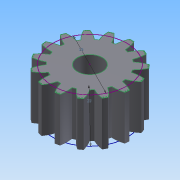
# Autodesk Inventor part: Spur Gear1
Saved by Autodesk Inventor 2015 (Build 190159000, 159)
## iProperties
Created: 2014-09-02
Part Number: Spur Gear1
Material: Steel
Document SubType Name: Modeling
Designer: shohei
Categories: <?xml version="1.0" encoding="UTF-16"?> <MemberInstance><Categories><FamilyTemplate><FamilyTemplateParameter ValueType="xs:double" Id="1" ObjectReferenceKey="da_z" ObjectType="kUserParameterObject"/><FamilyTemplateParameter ValueType="xs:double" Id="2" ObjectReferenceKey="da_b" ObjectType="kUserParameterObject"/><FamilyTemplateParameter ValueType="xs:double" Id="3" ObjectReferenceKey="da_beta" ObjectType="kUserParameterObject"/><FamilyTemplateParameter ValueType="xs:double" Id="4" ObjectReferenceKey="da_da" ObjectType="kUserParameterObject"/><FamilyTemplateParameter ValueType="xs:double" Id="5" ObjectReferenceKey="da_aw" ObjectType="kUserParameterObject"/><FamilyTemplateParameter ValueType="xs:string" Id="6" ObjectReferenceKey="EAIAABAAAACIAQAAAAAAAIAAAAAAAAAA" ObjectType="83910656" SubObjectId="SurfaceGeometry"/></FamilyTemplate><ParamToTemplateMap><ParamToTemplate CategoryParameter="//CategoryParameter[@InternalName='046C89C9-8512-4d59-83FE-43B91F4F132A']" TemplateParameter="1"/><ParamToTemplate CategoryParameter="//CategoryParameter[@InternalName='2552DF32-E462-4b46-AEBF-C6C7768E72AC']" TemplateParameter="2"/><ParamToTemplate CategoryParameter="//CategoryParameter[@InternalName='C9EE641D-15FC-4fae-A226-E94C4372FDD7']" TemplateParameter="3"/><ParamToTemplate><ParamToTemplate CategoryParameter="//CategoryParameter[@InternalName='00B6519A-459B-49c7-AD84-2E56D39A5744']" ConstantValue="0.000000"/></ParamToTemplate><ParamToTemplate><ParamToTemplate CategoryParameter="//CategoryParameter[@InternalName='04B31F0E-C7A6-4894-AA32-9629BEFACF47']" ConstantValue="1.000000"/></ParamToTemplate><ParamToTemplate><ParamToTemplate CategoryParameter="//CategoryParameter[@InternalName='43CBEC2E-7847-49e7-A936-2F7889FCB2D9']" ConstantValue="0.250000"/></ParamToTemplate><ParamToTemplate><ParamToTemplate CategoryParameter="//CategoryParameter[@InternalName='B1EFC894-105D-4ebd-86BF-FA20ED196853']" ConstantValue="0.350000"/></ParamToTemplate><ParamToTemplate><ParamToTemplate CategoryParameter="//CategoryParameter[@InternalName='51175063-3D10-4879-93E8-6246FE8B403D']" ConstantValue="2060000000.000000"/></ParamToTemplate><ParamToTemplate><ParamToTemplate CategoryParameter="//CategoryParameter[@InternalName='A3A52E27-4454-46a9-B0BD-C932399B70AF']" ConstantValue="0.300000"/></ParamToTemplate><ParamToTemplate><ParamToTemplate CategoryParameter="//CategoryParameter[@InternalName='91B76062-C214-41d9-B1B9-14D2AB99603D']" ConstantValue="0.100000"/></ParamToTemplate><ParamToTemplate><ParamToTemplate CategoryParameter="//CategoryParameter[@InternalName='374E806E-8B8A-4dda-A9AA-1039D6500AD2']" ConstantValue="10.000000"/></ParamToTemplate><ParamToTemplate><ParamToTemplate CategoryParameter="//CategoryParameter[@InternalName='2D373A89-B862-43d6-8D0B-0CBF12AB9F6C']" ConstantValue="0.349066"/></ParamToTemplate><ParamToTemplate CategoryParameter="//CategoryParameter[@InternalName='37777632-D6A2-4fac-9D53-DB8ACD95C989']" TemplateParameter="4"/><ParamToTemplate CategoryParameter="//CategoryParameter[@InternalName='FD1017F1-B727-4f7e-9707-0F86F1FF9423']" TemplateParameter="5"/><ParamToTemplate><ParamToTemplate CategoryParameter="//CategoryParameter[@InternalName='9E1B4470-B2D3-4ff1-B813-535BB4CDF51A']" ConstantValue="3520000.000000"/></ParamToTemplate><ParamToTemplate><ParamToTemplate CategoryParameter="//CategoryParameter[@InternalName='F8452263-BFF6-458c-9FB1-07C4B99E95CD']" ConstantValue="11400000.000000"/></ParamToTemplate><ParamToTemplate><ParamToTemplate CategoryParameter="//CategoryParameter[@InternalName='3E3BB259-FD49-497f-8171-6EBC954A3479']" ConstantValue="2.000000"/></ParamToTemplate><ParamToTemplate CategoryParameter="//CategoryParameter[@InternalName='27C3BAF2-7550-4e4b-AE2C-0DB134B7D9B7']" TemplateParameter="6"/></ParamToTemplateMap><Category DisplayName="Gear" InternalName="DC85795E-93AB-48d5-8EEE-5A27447B64BD" Mnemonic="Gear"><CategoryParameter DisplayName="z" InternalName="046C89C9-8512-4d59-83FE-43B91F4F132A" Mnemonic="z"/><CategoryParameter DisplayName="b" InternalName="2552DF32-E462-4b46-AEBF-C6C7768E72AC" Mnemonic="b"/><CategoryParameter DisplayName="||b|" InternalName="C9EE641D-15FC-4fae-A226-E94C4372FDD7" Mnemonic="beta"/><CategoryParameter DisplayName="x" InternalName="00B6519A-459B-49c7-AD84-2E56D39A5744" Mnemonic="x"/><CategoryParameter DisplayName="a*" InternalName="04B31F0E-C7A6-4894-AA32-9629BEFACF47" Mnemonic="a"/><CategoryParameter DisplayName="c*" InternalName="43CBEC2E-7847-49e7-A936-2F7889FCB2D9" Mnemonic="c"/><CategoryParameter DisplayName="r|.f|*" InternalName="B1EFC894-105D-4ebd-86BF-FA20ED196853" Mnemonic="rf"/><CategoryParameter DisplayName="E" InternalName="51175063-3D10-4879-93E8-6246FE8B403D" Mnemonic="E"/><CategoryParameter DisplayName="||m|" InternalName="A3A52E27-4454-46a9-B0BD-C932399B70AF" Mnemonic="mi"/><Category DisplayName="SpurGear" InternalName="26C5A22E-A91E-4dfd-A3B3-23CCAFAE1764" Mnemonic="SpurGear"><CategoryParameter DisplayName="m" InternalName="91B76062-C214-41d9-B1B9-14D2AB99603D" Mnemonic="m"/><CategoryParameter DisplayName="P" InternalName="374E806E-8B8A-4dda-A9AA-1039D6500AD2" Mnemonic="PP"/><CategoryParameter DisplayName="||a|" InternalName="2D373A89-B862-43d6-8D0B-0CBF12AB9F6C" Mnemonic="alpha"/><CategoryParameter DisplayName="d|.a|" InternalName="37777632-D6A2-4fac-9D53-DB8ACD95C989" Mnemonic="da"/><CategoryParameter DisplayName="a|.w|" InternalName="FD1017F1-B727-4f7e-9707-0F86F1FF9423" Mnemonic="aw"/><CategoryParameter DisplayName="||s||.Flim|" InternalName="9E1B4470-B2D3-4ff1-B813-535BB4CDF51A" Mnemonic="sFlim"/><CategoryParameter DisplayName="||s||.Hlim|" InternalName="F8452263-BFF6-458c-9FB1-07C4B99E95CD" Mnemonic="sHlim"/><CategoryParameter DisplayName="type" InternalName="3E3BB259-FD49-497f-8171-6EBC954A3479" Mnemonic="type"/><CategoryParameter DisplayName="PitchDiameter" InternalName="27C3BAF2-7550-4e4b-AE2C-0DB134B7D9B7" Mnemonic="IDS_PITCHDIAM"/></Category></Category></Categories></MemberInstance>
Density: 1 g/cm^3
Appearance: Steel
Author: shohei
Autodesk Inventor part; units mm, degrees
sketch "Sketch1" plane through (0, 0, 0) normal (0, 0, 1) x (1, 0, 0)
  circle A0 centre (0, 0) radius 8.5
  dimension "d0" = 17
  constraints: 1 centre point
  measures "d0" diameter of A0
extrude "Extrusion1" add sketch "Sketch1" along normal blind 9
ref_plane "Work Plane2" through (0, 0, 4.5) normal (0, 0, 1) x (1, 0, 0)
sketch "Sketch2" plane through (0, 0, 0) normal (0, 0, -1) x (-1, 0, 0)
  circle A0 centre (0, 0) radius 8.5 projected
  circle A1 centre (0, 0) radius 7.5
  dimension "d3" = 15
  constraints: 1 centre point, 1 coincident
  measures "d3" diameter of A1
surface extrude "Pitch Diameter" sketch "Sketch2" against normal through all shown no curves A1
ref_plane "Work Plane8" through (0, 0, 0) normal (0.9781476, 0.2079117, 0) x (0, 0, 1)
ref_plane "Work Plane9" through (0, 0, 0) normal (1, 0, 0) x (0, 1, 0)
spur gear teeth "Spur Gear" teeth 15 pitch diameter 15 tip diameter 17 root diameter 12.5 face width 20 start plane through (0, 0, 0) normal (0, 0, -1) x (-1, 0, 0)
sketch "Sketch3" plane through (0, 0, 9) normal (0, 0, 1) x (1, 0, 0)
  circle A0 centre (0, 0) radius 2.5
  dimension "d49" = 5
  constraints: 1 centre point, 1 coincident
  measures "d49" diameter of A0
extrude "Extrusion2" cut sketch "Sketch3" against normal through all
sketch "Sketch4" plane through (0, 0, 0) normal (0, 0, -1) x (-1, 0, 0)
  circle A0 centre (0, 0) radius 7.5
  dimension "d52" = 15
  constraints: 1 centre point, 1 coincident
  measures "d52" diameter of A0
sketch "Sketch5" plane through (0, 0, 9) normal (0, 0, 1) x (1, 0, 0)
  circle A0 centre (0, 0) radius 2.5 projected
  arc A1 (0.4449, 8.4884) -> (-0.4449, 8.4884) centre (0, 0) ccw projected
  arc A2 (-8.3954, -1.3297) -> (-6.037, -1.6176) centre (-6.3707, 5.4511) ccw projected
  arc A3 (-6.037, -1.6176) -> (-5.8349, -2.2398) centre (0, 0) ccw projected
  arc A4 (-5.8349, -2.2398) -> (-7.5736, -3.8589) centre (-1.9499, -8.1547) ccw projected
  arc A5 (-7.5736, -3.8589) -> (-7.1287, -4.6294) centre (0, 0) ccw projected
  arc A6 (-7.1287, -4.6294) -> (-4.8572, -3.9333) centre (-8.0371, 2.3886) ccw projected
  arc A7 (-4.8572, -3.9333) -> (-4.4194, -4.4194) centre (0, 0) ccw projected
  arc A8 (-4.4194, -4.4194) -> (-5.3492, -6.6057) centre (1.5354, -8.2428) ccw projected
  arc A9 (-5.3492, -6.6057) -> (-4.6294, -7.1287) centre (0, 0) ccw projected
  arc A10 (-4.6294, -7.1287) -> (-2.8374, -5.5688) centre (-8.3138, -1.0869) ccw projected
  arc A11 (-2.8374, -5.5688) -> (-2.2398, -5.8349) centre (0, 0) ccw projected
  arc A12 (-2.2398, -5.8349) -> (-2.2, -8.2104) centre (4.7554, -6.9056) ccw projected
  arc A13 (-2.2, -8.2104) -> (-1.3297, -8.3954) centre (0, 0) ccw projected
  arc A14 (-1.3297, -8.3954) -> (-0.3271, -6.2414) centre (-7.153, -4.3744) ccw projected
  arc A15 (-0.3271, -6.2414) -> (0.3271, -6.2414) centre (0, 0) ccw projected
  arc A16 (0.3271, -6.2414) -> (1.3297, -8.3954) centre (7.153, -4.3744) ccw projected
  arc A17 (1.3297, -8.3954) -> (2.2, -8.2104) centre (0, 0) ccw projected
  arc A18 (2.2, -8.2104) -> (2.2398, -5.8349) centre (-4.7554, -6.9056) ccw projected
  arc A19 (2.2398, -5.8349) -> (2.8374, -5.5688) centre (0, 0) ccw projected
  arc A20 (2.8374, -5.5688) -> (4.6294, -7.1287) centre (8.3138, -1.0869) ccw projected
  arc A21 (4.6294, -7.1287) -> (5.3492, -6.6057) centre (0, 0) ccw projected
  arc A22 (5.3492, -6.6057) -> (4.4194, -4.4194) centre (-1.5354, -8.2428) ccw projected
  arc A23 (4.4194, -4.4194) -> (4.8572, -3.9333) centre (0, 0) ccw projected
  arc A24 (4.8572, -3.9333) -> (7.1287, -4.6294) centre (8.0371, 2.3886) ccw projected
  arc A25 (7.1287, -4.6294) -> (7.5736, -3.8589) centre (0, 0) ccw projected
  arc A26 (7.5736, -3.8589) -> (5.8349, -2.2398) centre (1.9499, -8.1547) ccw projected
  arc A27 (5.8349, -2.2398) -> (6.037, -1.6176) centre (0, 0) ccw projected
  arc A28 (6.037, -1.6176) -> (8.3954, -1.3297) centre (6.3707, 5.4511) ccw projected
  arc A29 (8.3954, -1.3297) -> (8.4884, -0.4449) centre (0, 0) ccw projected
  arc A30 (8.4884, -0.4449) -> (6.2414, 0.3271) centre (5.0982, -6.6566) ccw projected
  arc A31 (6.2414, 0.3271) -> (6.1731, 0.9777) centre (0, 0) ccw projected
  arc A32 (6.1731, 0.9777) -> (8.2104, 2.2) centre (3.6028, 7.5711) ccw projected
  arc A33 (8.2104, 2.2) -> (7.9354, 3.0461) centre (0, 0) ccw projected
  arc A34 (7.9354, 3.0461) -> (5.5688, 2.8374) centre (7.3649, -4.0075) ccw projected
  arc A35 (5.5688, 2.8374) -> (5.2417, 3.404) centre (0, 0) ccw projected
  arc A36 (5.2417, 3.404) -> (6.6057, 5.3492) centre (0.2119, 8.3819) ccw projected
  arc A37 (6.6057, 5.3492) -> (6.0104, 6.0104) centre (0, 0) ccw projected
  arc A38 (6.0104, 6.0104) -> (3.9333, 4.8572) centre (8.3581, -0.6654) ccw projected
  arc A39 (3.9333, 4.8572) -> (3.404, 5.2417) centre (0, 0) ccw projected
  arc A40 (3.404, 5.2417) -> (3.8589, 7.5736) centre (-3.2157, 7.7434) ccw projected
  arc A41 (3.8589, 7.5736) -> (3.0461, 7.9354) centre (0, 0) ccw projected
  arc A42 (3.0461, 7.9354) -> (1.6176, 6.037) centre (7.9062, 2.7917) ccw projected
  arc A43 (1.6176, 6.037) -> (0.9777, 6.1731) centre (0, 0) ccw projected
  arc A44 (0.9777, 6.1731) -> (0.4449, 8.4884) centre (-6.0872, 5.766) ccw projected
  arc A45 (-0.4449, 8.4884) -> (-0.9777, 6.1731) centre (6.0872, 5.766) ccw projected
  arc A46 (-0.9777, 6.1731) -> (-1.6176, 6.037) centre (0, 0) ccw projected
  arc A47 (-1.6176, 6.037) -> (-3.0461, 7.9354) centre (-7.9062, 2.7917) ccw projected
  circle A48 centre (0, 0) radius 7.5
  arc A49 (-3.8589, 7.5736) -> (-3.404, 5.2417) centre (3.2157, 7.7434) ccw projected
  arc A50 (-3.404, 5.2417) -> (-3.9333, 4.8572) centre (0, 0) ccw projected
  arc A51 (-3.9333, 4.8572) -> (-6.0104, 6.0104) centre (-8.3581, -0.6654) ccw projected
  arc A52 (-6.0104, 6.0104) -> (-6.6057, 5.3492) centre (0, 0) ccw projected
  arc A53 (-6.6057, 5.3492) -> (-5.2417, 3.404) centre (-0.2119, 8.3819) ccw projected
  arc A54 (-5.2417, 3.404) -> (-5.5688, 2.8374) centre (0, 0) ccw projected
  arc A55 (-5.5688, 2.8374) -> (-7.9354, 3.0461) centre (-7.3649, -4.0075) ccw projected
  arc A56 (-7.9354, 3.0461) -> (-8.2104, 2.2) centre (0, 0) ccw projected
  arc A57 (-8.2104, 2.2) -> (-6.1731, 0.9777) centre (-3.6028, 7.5711) ccw projected
  arc A58 (-6.1731, 0.9777) -> (-6.2414, 0.3271) centre (0, 0) ccw projected
  arc A59 (-6.2414, 0.3271) -> (-8.4884, -0.4449) centre (-5.0982, -6.6566) ccw projected
  arc A60 (-8.4884, -0.4449) -> (-8.3954, -1.3297) centre (0, 0) ccw projected
  arc A61 (-3.0461, 7.9354) -> (-3.8589, 7.5736) centre (0, 0) ccw projected
  dimension "d53" = 15
  constraints: 1 centre point
  measures "d53" diameter of A48
equation "\"d0\" = da_da"
equation "\"d3\" = da_dw"
equation "\"d16\" = da_aw"
equation "\"d43\" = da_aw"
equation "\"d46\" = da_aw"
equation "\"da_da\" = 17"
equation "\"da_dw\" = 15"
equation "\"da_aw\" = 15"
body "Solid1"
body "Srf1"
